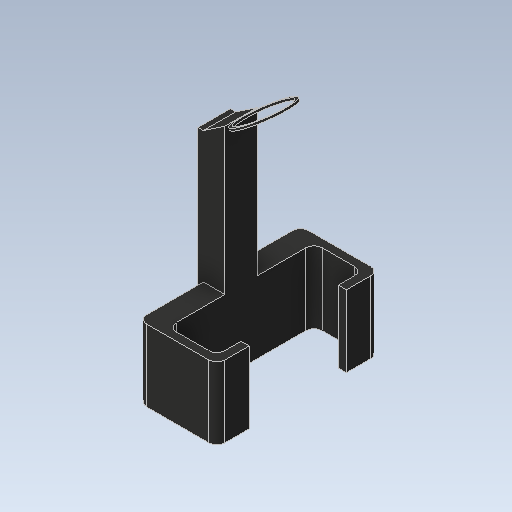
# Autodesk Inventor part: TRUNK_1
Saved by Autodesk Inventor 2021 (Build 250183000, 183)
## iProperties
Created: 2021-03-14
Part Number: TRUNK_1
Material: Rubber, Silicone
Document SubType Name: Modeling
Designer: 91760
Density: 1.25 g/cm^3
Appearance: Rubber - Black
Author: 91760
Autodesk Inventor part; units mm, degrees
ref_plane "YZ Plane" through (0, 0, 0) normal (1, 0, 0) x (0, 1, 0)
ref_plane "XZ Plane" through (0, 0, 0) normal (0, 1, 0) x (-1, 0, 0)
ref_plane "XY Plane" through (0, 0, 0) normal (0, 0, 1) x (1, 0, 0)
sketch "Sketch1" plane through (0, 0, 0) normal (0, 0, 1) x (1, 0, 0)
  line L0 (0, -27) -> (0, 396)
  line L1 (0, -27) -> (40, -27)
  line L2 (40, -27) -> (40, 423)
  line L3 (40, 423) -> (0, 396)
  point P0 (0, 0)
  dimension "d0" = 423
  dimension "d1" = 27
  dimension "d2" = 40
  dimension "d3" = 450
  constraints: 8 end point, 2 vertical, 1 horizontal, 1 perpendicular
  measures "d0" distance of L0.start L0.end
  measures "d1" distance of point (0, 0) L0.start
  measures "d2" distance of L0.start L1.end
  measures "d3" distance of L1.end L2.end
extrude "Extrusion1" add sketch "Sketch1" along normal mid plane 300
sketch "Sketch2" plane through (40, -27, 150) normal (1, 0, 0) x (0, 0, -1)
  line L0 (0, 450) -> (300, 450) construction
  line L1 (150, 450) -> (150, 0) construction
  line L2 (300, 0) -> (0, 0) construction
  line L3 (120, 450) -> (120, 180)
  line L4 (120, 180) -> (0, 180)
  line L5 (0, 180) -> (0, 450)
  line L6 (0, 423) -> (0, 0) projected
  line L7 (300, 450) -> (0, 450) construction
  line L8 (180, 450) -> (180, 180)
  line L9 (180, 180) -> (300, 180)
  line L10 (300, 180) -> (300, 450)
  line L11 (0, 0) -> (0, 450) projected
  line L12 (0, 450) -> (120, 450)
  line L13 (180, 450) -> (300, 450)
  point P0 (150, 27)
  dimension "d6" = 270
  constraints: 20 end point, 5 symmetric about line, 3 perpendicular, 2 midpoint, 2 point on line, 1 collinear, 1 parallel, 1 vertical
  measures "d6" distance of L3.start L3.end
extrude "Extrusion2" cut sketch "Sketch2" against normal blind 263.525
sketch "Sketch3" plane through (0, 0, 150) normal (0, 0, 1) x (1, 0, 0)
  line L0 (40, -27) -> (0, -27) projected
  arc A0 (27, -27) -> (0, 0) centre (0, -27) ccw
  line L1 (0, -27) -> (0, 153) projected
  line L2 (0, 0) -> (0, -27)
  line L3 (0, -27) -> (27, -27)
  dimension "d9" = 27
  constraints: 4 end point, 2 collinear, 2 point on circle, 1 centre point, 1 point on line
  measures "d9" radius of A0
extrude "Extrusion3" cut sketch "Sketch3" against normal blind 400
sketch "Sketch4" plane through (40, -27, 150) normal (1, 0, 0) x (0, 0, -1)
  line L0 (0, 0) -> (300, 0) projected
  line L1 (0, 0) -> (120, 0)
  line L2 (120, 0) -> (120, 27)
  line L3 (300, 27) -> (0, 27) projected
  line L4 (120, 27) -> (0, 27)
  line L5 (0, 0) -> (0, 180) projected
  line L6 (0, 27) -> (0, 0)
  point P0 (150, 27)
  dimension "d12" = 120
  dimension "d13" = 27
  constraints: 8 end point, 2 point on line, 1 collinear
  measures "d12" distance of L0.start L1.end
  measures "d13" distance of L1.end L2.end
extrude "Extrusion4" cut sketch "Sketch4" against normal blind 400
mirror "Mirror1" about plane through (0, 0, 0) normal (0, 0, 1) of "Extrusion4"
sketch "Sketch5" plane through (40, 153, 150) normal (0, 1, 0) x (1, 0, 0)
  point P0 (-40, 150)
sketch "Sketch6" plane through (40, 423, 30) normal (-0.5594729, 0.8288487, 0) x (0.8288487, 0.5594729, 0)
  line L0 (0, 0) -> (0, 60) projected
  line L1 (0, 30) -> (50, 30)
  circle A0 centre (50, 30) radius 50
  circle A1 centre (50, 30) radius 45
  point P0 (-269.811, 30)
  dimension "d16" = 50
  dimension "d17" = 90
  constraints: 2 coincident, 2 end point, 1 centre point, 1 horizontal, 1 horizontal alignment, 1 midpoint, 2 other
  measures "d16" distance of L1.start L1.end
  measures "d17" diameter of A1
extrude "Extrusion5" add sketch "Sketch6" against normal blind 4
sketch "Sketch7" plane through (40, 153, -30) normal (1, 0, 0) x (0, 0, -1)
  line L0 (-60, -153) -> (-60, -180) projected
  line L1 (-60, -153) -> (-60, -133)
  line L2 (-60, -133) -> (-180, -133)
  line L3 (-180, -153) -> (-180, 0) projected
  line L4 (-180, -153) -> (-60, -153) projected
  line L5 (-180, -153) -> (-60, -153)
  point P0 (-30, -153)
  dimension "d20" = 20
  constraints: 6 end point, 1 horizontal, 1 perpendicular, 1 point on line, 1 vertical
  measures "d20" distance of L0.start L1.end
extrude "Extrusion6" cut sketch "Sketch7" against normal blind 300
mirror "Mirror2" about plane through (0, 0, 0) normal (0, 0, 1) of "Extrusion6"
sketch "Sketch8" plane through (0, 0, 150) normal (0, 0, 1) x (1, 0, 0)
  point P0 (0, 0)
sketch "Sketch9" plane through (0, 0, 150) normal (0, 0, 1) x (1, 0, 0)
  point P0 (0, 0)
sketch "Sketch10" plane through (0, 0, 150) normal (0, 0, 1) x (1, 0, 0)
  point P0 (0, 0)
sketch "Sketch11" plane through (0, 0, 150) normal (0, 0, 1) x (1, 0, 0)
  line L0 (40, 153) -> (0, 153) projected
  line L1 (40, 20) -> (40, -27) projected
  line L2 (40, 153) -> (40, 20)
  line L3 (40, 20) -> (130, 20)
  line L4 (130, 20) -> (130, 153)
  line L5 (130, 153) -> (40, 153)
  point P0 (0, 0)
  dimension "d23" = 90
  constraints: 8 end point, 3 perpendicular, 1 vertical
  measures "d23" distance of L1.start L3.end
extrude "Extrusion7" add sketch "Sketch11" against normal blind 15
mirror "Mirror3" about plane through (0, 0, 0) normal (0, 0, 1) of "Extrusion7"
sketch "Sketch12" plane through (130, 20, 150) normal (1, 0, 0) x (0, 0, -1)
  line L0 (0, 133) -> (0, 0) projected
  line L1 (0, 133) -> (60, 133)
  line L2 (0, 133) -> (120, 133) projected
  line L3 (60, 133) -> (60, 0)
  line L4 (15, 0) -> (120, 0) projected
  line L5 (60, 0) -> (0, 0)
  line L6 (0, 0) -> (0, 133)
  point P0 (150, -20)
  constraints: 8 end point, 2 perpendicular, 1 horizontal, 1 midpoint, 1 point on line
extrude "Extrusion8" add sketch "Sketch12" along normal blind 15
mirror "Mirror4" about plane through (0, 0, 0) normal (0, 0, 1) of "Extrusion8"
sketch "Sketch13" plane through (40, 153, -30) normal (1, 0, 0) x (0, 0, -1)
  line L0 (-60, -153) -> (-60, -133) projected
  line L1 (-60, -133) -> (-40, -133)
  line L2 (-40, -133) -> (-40, -180)
  line L3 (-60, -180) -> (0, -180) projected
  line L4 (-40, -180) -> (-60, -180)
  line L5 (-60, -180) -> (-60, -133)
  point P0 (-30, -153)
  dimension "d28" = 20
  constraints: 8 end point, 2 horizontal, 2 perpendicular, 1 point on line
  measures "d28" distance of L0.end L1.end
extrude "Extrusion9" cut sketch "Sketch13" against normal blind 200
mirror "Mirror5" about plane through (0, 0, 0) normal (0, 0, 1) of "Extrusion9"
sketch "Sketch14" plane through (0, 153, 30) normal (0, 1, 0) x (1, 0, 0)
  line L0 (0, -120) -> (0, 0) projected
  line L1 (0, 0) -> (0, -105)
  line L2 (145, -120) -> (0, -120) projected
  line L3 (15, -120) -> (145, -120)
  arc A0 (0, -105) -> (15, -120) centre (15, -105) ccw
  line L4 (0, 0) -> (0, -120)
  line L5 (0, -120) -> (145, -120)
  arc A1 (0, -105) -> (15, -120) centre (15, -105) ccw
  line L6 (0, -105) -> (0, -120)
  line L7 (0, -120) -> (15, -120)
  arc A2 (0, -105) -> (15, -120) centre (15, -105) ccw
  point P0 (0, 30)
  dimension "d31" = 15
  constraints: 12 end point, 7 point on circle, 6 collinear, 4 tangent, 3 centre point, 3 point on line, 2 coincident
  measures "d31" radius of A0
extrude "Extrusion10" cut sketch "Sketch14" against normal blind 200
sketch "Sketch15" plane through (0, 153, 30) normal (0, 1, 0) x (1, 0, 0)
  line L0 (40, 0) -> (40, -105) projected
  line L1 (40, 0) -> (40, -90)
  line L2 (40, -105) -> (130, -105) projected
  line L3 (55, -105) -> (130, -105)
  arc A0 (40, -90) -> (55, -105) centre (55, -90) ccw
  arc A1 (40, -90) -> (55, -105) centre (55, -90) ccw
  line L4 (40, -90) -> (40, -105)
  line L5 (40, -105) -> (55, -105)
  point P0 (0, 30)
  dimension "d34" = 15
  constraints: 8 end point, 4 point on circle, 4 tangent, 3 collinear, 2 centre point, 2 point on line, 1 coincident, 1 perpendicular
  measures "d34" radius of A0
sketch "Sketch16" plane through (0, 0, 150) normal (0, 0, 1) x (1, 0, 0)
  point P0 (0, 0)
extrude "Extrusion11" add sketch "Sketch15" against normal blind 133
mirror "Mirror6" about plane through (0, 0, 0) normal (0, 0, 1) of "Extrusion11", "Extrusion10"
sketch "Sketch17" plane through (0, 153, 30) normal (0, 1, 0) x (1, 0, 0)
  line L0 (130, -60) -> (130, -105) projected
  line L1 (130, -60) -> (130, -90)
  line L2 (55, -105) -> (130, -105) projected
  line L3 (115, -105) -> (55, -105)
  arc A0 (115, -105) -> (130, -90) centre (115, -90) ccw
  arc A1 (115, -105) -> (130, -90) centre (115, -90) ccw
  line L4 (130, -90) -> (130, -105)
  line L5 (130, -105) -> (115, -105)
  point P0 (0, 30)
  dimension "d37" = 15
  constraints: 8 end point, 6 tangent, 4 point on circle, 2 centre point, 2 collinear, 1 coincident, 1 perpendicular, 1 vertical
  measures "d37" radius of A0
extrude "Extrusion12" add sketch "Sketch17" against normal blind 133
mirror "Mirror7" about plane through (0, 0, 0) normal (0, 0, 1) of "Extrusion12"
sketch "Sketch18" plane through (0, 153, -30) normal (0, 1, 0) x (1, 0, 0)
  line L0 (15, 120) -> (145, 120) projected
  line L1 (15, 120) -> (130, 120)
  line L2 (145, 120) -> (145, 60) projected
  line L3 (145, 105) -> (145, 60)
  arc A0 (145, 105) -> (130, 120) centre (130, 105) ccw
  arc A1 (145, 105) -> (130, 120) centre (130, 105) ccw
  line L4 (130, 120) -> (145, 120)
  line L5 (145, 120) -> (145, 105)
  point P0 (0, -30)
  dimension "d40" = 15
  constraints: 8 end point, 4 point on circle, 3 collinear, 3 tangent, 2 centre point, 2 point on line, 1 coincident, 1 horizontal
  measures "d40" radius of A0
extrude "Extrusion13" cut sketch "Sketch18" against normal blind 133
mirror "Mirror8" about plane through (0, 0, 0) normal (0, 0, 1) of "Extrusion13"
scale "Scale1" factors (2, 2, 2) then translate (0, -153, -30) bodies 1
sketch "Sketch19" plane through (80, 153, 30) normal (0, 0, 1) x (1, 0, 0)
  point P0 (-80, -153)
sketch "Sketch20" plane through (80, -207, -10) normal (0, 0, 1) x (1, 0, 0)
  point P0 (-80, 207)
sketch "Sketch21" plane through (80, -207, -10) normal (0, 0, 1) x (1, 0, 0)
  point P0 (-80, 207)
sketch "Sketch22" plane through (80, 153, 30) normal (0, 0, 1) x (1, 0, 0)
  line L0 (0, 540) -> (-80, 486) projected
  line L1 (-80, 486) -> (-80, -360)
  line L2 (-80, -360) -> (-100, -360)
  line L3 (-100, -360) -> (-100, 486)
  line L4 (-100, 486) -> (-80, 486)
  point P0 (-80, -153)
  dimension "d46" = 846
  dimension "d47" = 20
  constraints: 8 end point, 3 perpendicular, 1 vertical
  measures "d46" distance of L0.end L1.end
  measures "d47" distance of L1.end L2.end
sketch "Sketch23" plane through (0, 153, 30) normal (-1, 0, 0) x (0, 0, 1)
  point P0 (-30, -153)
extrude "Extrusion14" add sketch "Sketch22" against normal blind 129
sketch "Sketch24" plane through (0, -207, 30) normal (1, 0, 0) x (0, 0, -1)
  line L0 (40, 94) -> (40, 0) projected
  line L1 (40, 94) -> (40, 0)
  line L2 (0, 0) -> (0, 846) projected
  line L3 (40, 0) -> (0, 0)
  line L4 (0, 0) -> (0, 94)
  line L5 (0, 94) -> (40, 94)
  line L6 (40, 0) -> (0, 0)
  point P0 (30, 207)
  constraints: 10 end point, 2 equal length, 1 horizontal, 1 perpendicular, 1 point on line
extrude "Extrusion15" cut sketch "Sketch24" against normal blind 129
sketch "Sketch25" plane through (0, -207, -99) normal (1, 0, 0) x (0, 0, -1)
  line L0 (0, 94) -> (-49, 94) projected
  line L1 (-49, 94) -> (0, 94)
  line L2 (0, 0) -> (0, 846) projected
  line L3 (0, 94) -> (0, 0)
  line L4 (0, 0) -> (-44.5, 0)
  line L5 (-89, 0) -> (0, 0) projected
  line L6 (-49, 0) -> (-49, 54) projected
  line L7 (-49, 0) -> (-49, 94)
  point P0 (-99, 207)
  constraints: 8 end point, 2 collinear, 1 horizontal, 1 midpoint
extrude "Extrusion16" cut sketch "Sketch25" against normal blind 129
sketch "Sketch26" plane through (80, -207, -10) normal (0, 0, 1) x (1, 0, 0)
  line L0 (-100, 0) -> (-100, 94) projected
  line L1 (-26, 0) -> (0, 0) projected
  arc A0 (-26, 0) -> (-100, 74) centre (-100, 0) ccw
  line L2 (-100, 0) -> (-26, 0)
  line L3 (-100, 0) -> (-100, 74)
  line L4 (0, 94) -> (-100, 94) projected
  point P0 (-80, 207)
  constraints: 4 end point, 2 point on circle, 1 centre point, 1 horizontal, 1 perpendicular
extrude "Extrusion17" cut sketch "Sketch26" against normal blind 129
sketch "Sketch27" plane through (0, 153, -90) normal (1, 0, 0) x (0, 0, -1)
  line L0 (-120, 486) -> (9, 486) projected
  line L1 (9, 486) -> (9, 0)
  line L2 (9, -266) -> (9, 486) projected
  line L3 (0, 486) -> (0, 0) projected
  line L4 (9, 0) -> (0, 0)
  line L5 (0, 0) -> (0, 486)
  line L6 (0, 486) -> (9, 486)
  point P0 (-90, -153)
  constraints: 8 end point, 2 perpendicular, 1 collinear, 1 point on line
extrude "Extrusion18" cut sketch "Sketch27" against normal blind 129
sketch "Sketch28" plane through (80, -207, -10) normal (0, 0, 1) x (1, 0, 0)
  line L0 (0, 0) -> (-26, 0) projected
  arc A0 (-10, 0) -> (-100, 90) centre (-100, 0) ccw
  line L1 (-10, 0) -> (-100, 0)
  line L2 (-100, 0) -> (-100, 90)
  point P0 (-80, 207)
  dimension "d58" = 90
  constraints: 4 end point, 2 point on circle, 1 centre point, 1 horizontal, 1 perpendicular, 1 point on line
  measures "d58" radius of A0
sketch "Sketch29" plane through (-20, -113, 30) normal (-1, 0, 0) x (0, 0, 1)
  point P0 (-30, 113)
sketch "Sketch30" plane through (80, -207, -10) normal (0, 0, 1) x (1, 0, 0)
  line L0 (-100, 74) -> (-100, 94) projected
  line L1 (-100, 74) -> (0, 74)
  line L2 (0, 94) -> (0, 0) projected
  line L3 (0, 74) -> (0, 0)
  line L4 (0, 0) -> (0, -50)
  line L5 (0, -50) -> (-100, -50)
  line L6 (-100, -50) -> (-100, 74)
  point P0 (-80, 207)
  dimension "d59" = 50
  constraints: 10 end point, 2 perpendicular, 2 point on line, 1 collinear, 1 horizontal
  measures "d59" distance of L2.end L4.end
extrude "Extrusion19" add sketch "Sketch30" against normal blind 40
sketch "Sketch31" plane through (-20, -113, -10) normal (0, 0, 1) x (1, 0, 0)
  line L0 (100, -144) -> (0, -144) projected
  arc A0 (40, -144) -> (0, -104) centre (0, -144) ccw
  line L1 (0, -144) -> (0, 0) projected
  line L2 (0, -144) -> (40, -144)
  line L3 (0, -144) -> (0, -104)
  point P0 (20, 113)
  dimension "d62" = 40
  constraints: 4 end point, 2 point on circle, 1 centre point, 1 collinear, 1 perpendicular, 1 point on line
  measures "d62" radius of A0
extrude "Extrusion20" cut sketch "Sketch31" against normal blind 40
sketch "Sketch32" plane through (-20, -113, -10) normal (0, 0, 1) x (1, 0, 0)
  line L0 (100, -144) -> (40, -144) projected
  arc A0 (90, -144) -> (0, -54) centre (0, -144) ccw
  line L1 (0, -144) -> (90, -144)
  line L2 (0, -144) -> (0, -54)
  line L3 (0, -104) -> (0, 0) projected
  point P0 (20, 113)
  dimension "d65" = 90
  constraints: 4 end point, 2 collinear, 2 point on circle, 1 centre point, 1 point on line
  measures "d65" radius of A0
extrude "Extrusion21" add sketch "Sketch32" along normal blind 20
sketch "Sketch33" plane through (80, -113, -50) normal (0, 0, -1) x (-1, 0, 0)
  line L0 (100, -144) -> (10, -144) projected
  arc A0 (100, -54) -> (10, -144) centre (100, -144) ccw projected
  arc A1 (100, -54) -> (10, -144) centre (100, -144) ccw
  line L1 (100, -54) -> (100, -144)
  line L2 (100, -144) -> (10, -144)
  point P0 (80, 113)
  dimension "d68" = 90
  constraints: 4 end point, 2 point on circle, 1 centre point, 1 perpendicular, 1 vertical
  measures "d68" radius of A1
extrude "Extrusion22" add sketch "Sketch33" along normal blind 20
sketch "Sketch34" plane through (0, 153, 30) normal (0, 1, 0) x (1, 0, 0)
  point P0 (0, 30)
sketch "Sketch35" plane through (260, 153, -210) normal (0, 1, 0) x (1, 0, 0)
  point P0 (-260, -210)
body "Solid1"
